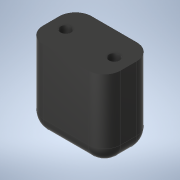
# Autodesk Inventor part: door_parts
Saved by Autodesk Inventor 2021.3 (Build 253353000, 353)
## iProperties
Created: 2019-07-23
Part Number: door_parts
Material: PAEK 樹脂
Document SubType Name: Modeling
Designer: gisen
Density: 1.32 g/cm^3
Appearance: 滑らか - 白
Author: gisen
Autodesk Inventor part; units mm, degrees
ref_plane "YZ Plane" through (0, 0, 0) normal (1, 0, 0) x (0, 1, 0)
ref_plane "XZ Plane" through (0, 0, 0) normal (0, 1, 0) x (-1, 0, 0)
ref_plane "XY Plane" through (0, 0, 0) normal (0, 0, 1) x (1, 0, 0)
sketch "スケッチ1" plane through (0, 0, 0) normal (0, 0, 1) x (1, 0, 0)
  line L0 (-26.4547, 10.8836) -> (-2.4547, 10.8836)
  line L1 (-2.4547, 10.8836) -> (-2.4547, -14.1164)
  line L2 (-2.4547, -14.1164) -> (-26.4547, -14.1164)
  line L3 (-26.4547, -14.1164) -> (-26.4547, 10.8836)
  point P0 (0, 0)
  dimension "d0" = 25
  dimension "d1" = 24
  constraints: 8 end point, 2 parallel, 1 horizontal, 1 perpendicular
  measures "d0" distance of L2.end L0.start
  measures "d1" distance of L0.start L0.end
extrude "押し出し1" add sketch "スケッチ1" along normal blind 15
sketch "スケッチ3" plane through (0, 0, 0) normal (0, 0, -1) x (-1, 0, 0)
  circle A0 centre (10.4547, -3.5864) radius 5
  line L0 (26.4547, 10.8836) -> (2.4547, 10.8836) projected
  line L1 (2.4547, 10.8836) -> (2.4547, -14.1164) projected
  point P0 (0, 0)
  dimension "d7" = 10
  dimension "d8" = 14.47
  dimension "d9" = 8
  constraints: 1 centre point
  measures "d7" diameter of A0
  measures "d8" distance from line of L0 A0.centre
  measures "d9" distance from line of L1 A0.centre
extrude "押し出し2" cut sketch "スケッチ3" against normal blind 10
fillet "フィレット1" radius 5 8 edges at (-2.4547, -14.1164, 7.5) (-14.4547, -14.1164, 15) (-14.4547, -14.1164, 0) (-26.4547, -1.6164, 15) (-26.4547, -14.1164, 7.5) (-26.4547, -1.6164, 0) (-2.4547, -1.6164, 15) (-2.4547, -1.6164, 0)
sketch "スケッチ4" plane through (-21.4547, 10.8836, 0) normal (0, 1, 0) x (1, 0, 0)
  arc A0 (19, -5) -> (14, 0) centre (14, -5) ccw projected
  line L0 (0, 0) -> (14, 0) projected
  arc A1 (0, 0) -> (-5, -5) centre (0, -5) ccw projected
  line L1 (-5, -5) -> (-5, -10) projected
  arc A2 (-5, -10) -> (0, -15) centre (0, -10) ccw projected
  line L2 (14, -15) -> (0, -15) projected
  arc A3 (14, -15) -> (19, -10) centre (14, -10) ccw projected
  line L3 (19, -5) -> (19, -10) projected
  circle A4 centre (14.5, -7.5) radius 1.65
  circle A5 centre (-0.5, -7.5) radius 1.65
  point P0 (21.4547, 0)
  dimension "d13" = 3.3
  dimension "d14" = 4.5
  dimension "d15" = 7.5
  dimension "d22" = 15
  dimension "d23" = 3.3
  dimension "d24" = 7.5
  constraints: 2 centre point
  measures "d13" diameter of A4
  measures "d14" distance from line of L3 A4.centre
  measures "d15" distance from line of L0 A4.centre
  measures "d22" distance of A5.centre A4.centre
  measures "d23" diameter of A5
  measures "d24" distance from line of L0 A5.centre
extrude "押し出し3" cut sketch "スケッチ4" against normal blind 7 contours A4 | A5
